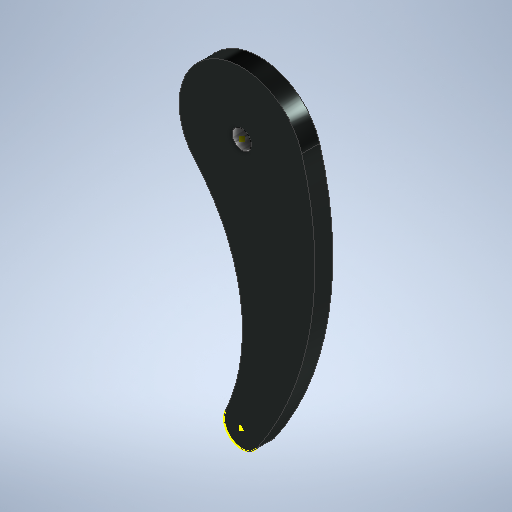
# Autodesk Inventor part: shooter
Saved by Autodesk Inventor 2025.4 (Build 294407000, 407)
## iProperties
Created: 2026-02-28
Part Number: shooter
Material: Polystyrene, Expanded
Document SubType Name: Modeling
Designer: youse
Density: 0.05 g/cm^3
Appearance: Chrome - Polished
Author: youse
## iProperties of the stored document shooter_3DPrint.ipt
Created: 2026-03-12
Part Number: shooter_3DPrint
Material: Generic
Document SubType Name: Modeling
Designer: youse
Density: 1 g/cm^3
Appearance: Default
Author: youse
Autodesk Inventor part; units mm, degrees
ref_plane "YZ Plane" through (0, 0, 0) normal (1, 0, 0) x (0, 1, 0)
ref_plane "XZ Plane" through (0, 0, 0) normal (0, 1, 0) x (-1, 0, 0)
ref_plane "XY Plane" through (0, 0, 0) normal (0, 0, 1) x (1, 0, 0)
sketch "Sketch1" plane through (0, 0, 0) normal (0, 0, 1) x (1, 0, 0)
  arc A0 (16.7907, 4.9318) -> (-13.022, -11.6909) centre (0, 0) ccw
  arc A1 (-4.5405, -67.9061) -> (4.1009, -72.8606) centre (0, -70) ccw
  arc A2 (4.1009, -72.8606) -> (16.7907, 4.9318) centre (-70.6155, -20.7413) ccw
  arc A3 (-4.5405, -67.9061) -> (-13.022, -11.6909) centre (-51.5111, -46.2455) ccw
  dimension "d0" = 35
  dimension "d1" = 10
  dimension "d2" = 70
  dimension "d3" = 182.1971
  dimension "d7" = 103.4491
  constraints: 8 point on circle, 4 centre point, 4 tangent, 1 coincident, 1 vertical alignment
  measures "d0" diameter of A0
  measures "d1" diameter of A1
  measures "d2" distance of A1.centre point (0, 0)
  measures "d3" diameter of A2
  measures "d7" diameter of A3
extrude "Extrusion1" add sketch "Sketch1" along normal blind 5
sketch "Sketch2" plane through (0, 0, 5) normal (0, 0, 1) x (1, 0, 0)
  circle A0 centre (0, 0) radius 2.7
  dimension "d8" = 5.4
  constraints: 1 centre point, 1 coincident
  measures "d8" diameter of A0
extrude "Extrusion2" cut sketch "Sketch2" against normal through all
sketch "Sketch3" plane through (0, 0, 5) normal (0, 0, 1) x (1, 0, 0)
  arc A0 (-4.5405, -67.9061) -> (4.1009, -72.8606) centre (0, -70) ccw projected
  point P0 (0, 0)
body "Solid1"
